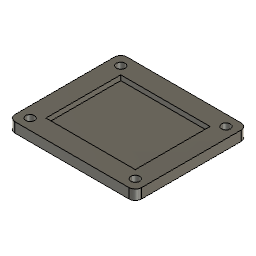
air_quality_sensor_holder (Autodesk Fusion 360 design; units mm, degrees)
Autodesk Fusion 360 part; units mm, degrees
sketch "Sketch10" plane through (0, 0, 0) normal (0, 0, 1) x (1, 0, 0)
  line L0 (0, 0) -> (45.72, 0)
  arc A0 (48.26, -2.54) -> (45.72, 0) centre (45.72, -2.54) ccw
  line L1 (45.72, -2.54) -> (48.26, -2.54) construction
  line L2 (45.72, -2.54) -> (45.72, 0) construction
  line L3 (48.26, -2.54) -> (48.26, -42.4361)
  arc A1 (48.26, -2.54) -> (45.72, 0) centre (45.72, -2.54) ccw
  arc A2 (45.72, -44.9761) -> (48.26, -42.4361) centre (45.72, -42.4361) ccw
  line L4 (0, -42.4361) -> (-2.54, -42.4361) construction
  line L5 (45.72, -44.9761) -> (0, -44.9761)
  arc A3 (-2.54, -42.4361) -> (0, -44.9761) centre (0, -42.4361) ccw
  arc A4 (-2.54, -42.4361) -> (0, -44.9761) centre (0, -42.4361) ccw
  line L6 (0, -42.4361) -> (0, -44.9761) construction
  arc A5 (0, 0) -> (-2.54, -2.54) centre (0, -2.54) ccw
  line L7 (-2.54, -42.4361) -> (-2.54, -2.54)
  point P0 (45.72, -44.9761)
  dimension "d5" = 45.72
  dimension "d7" = 2.54
  dimension "d8" = 90
  dimension "d9" = 39.8961
  dimension "d10" = 2.54
  dimension "d11" = 2.54
  dimension "d12" = 45.72
  dimension "d13" = 2.54
  dimension "d14" = 90
  dimension "d15" = 39.8961
  dimension "d16" = 2.54
  dimension "d17" = 2.54
  constraint coincident L0.start A5.start
  constraint horizontal L0
  constraint perpendicular L1 L3
  constraint coincident P0 A2.start
  constraint perpendicular L4 L7
  measures "d5" distance of L0.start L0.end
  measures "d7" radius of A0
  measures "d8" angle of L1 L2
  measures "d9" distance of A0.start L3.end
  measures "d10" radius of A1
  measures "d11" radius of A2
  measures "d12" distance of P0 L5.end
  measures "d13" radius of A4
  measures "d14" angle of L4 L6
  measures "d15" distance of L4.end A5.end
  measures "d16" radius of A3
  measures "d17" radius of A5
extrude "Extrude3" add sketch "Sketch10" along normal blind 4
sketch "Sketch11" plane through (0, 0, 4) normal (0, 0, 1) x (-1, 0, 0)
  arc A0 (-45.72, 44.9761) -> (-48.26, 42.4361) centre (-45.72, 42.4361) ccw
  line L0 (-48.26, 42.4361) -> (-48.26, 2.54)
  arc A1 (-48.26, 2.54) -> (-45.72, 0) centre (-45.72, 2.54) ccw
  line L1 (-45.72, 0) -> (0, 0)
  arc A2 (0, 0) -> (2.54, 2.54) centre (0, 2.54) ccw
  line L2 (2.54, 2.54) -> (2.54, 42.4361)
  arc A3 (2.54, 42.4361) -> (0, 44.9761) centre (0, 42.4361) ccw
  line L3 (0, 44.9761) -> (-45.72, 44.9761)
  circle A4 centre (-1.778, 4.318) radius 1.75
  dimension "d22" = 3.5
  measures "d22" diameter of A4
extrude "Extrude4" cut sketch "Sketch11" against normal blind 4 contours A4
sketch "Sketch12" plane through (0, 0, 4) normal (0, 0, 1) x (-1, 0, 0)
  circle A0 centre (-1.778, 4.318) radius 1.75
  arc A1 (-45.72, 44.9761) -> (-48.26, 42.4361) centre (-45.72, 42.4361) ccw
  line L0 (-48.26, 42.4361) -> (-48.26, 2.54)
  arc A2 (-48.26, 2.54) -> (-45.72, 0) centre (-45.72, 2.54) ccw
  line L1 (-45.72, 0) -> (0, 0)
  arc A3 (0, 0) -> (2.54, 2.54) centre (0, 2.54) ccw
  line L2 (2.54, 2.54) -> (2.54, 42.4361)
  arc A4 (2.54, 42.4361) -> (0, 44.9761) centre (0, 42.4361) ccw
  line L3 (0, 44.9761) -> (-45.72, 44.9761)
  circle A5 centre (-43.942, 4.318) radius 1.75
  dimension "d27" = 3.5
  measures "d27" diameter of A5
extrude "Extrude5" cut sketch "Sketch12" against normal blind 4 contours A5
sketch "Sketch13" plane through (0, 0, 4) normal (0, 0, 1) x (-1, 0, 0)
  circle A0 centre (-43.942, 4.318) radius 1.75
  circle A1 centre (-1.778, 4.318) radius 1.75
  arc A2 (-45.72, 44.9761) -> (-48.26, 42.4361) centre (-45.72, 42.4361) ccw
  line L0 (-48.26, 42.4361) -> (-48.26, 2.54)
  arc A3 (-48.26, 2.54) -> (-45.72, 0) centre (-45.72, 2.54) ccw
  line L1 (-45.72, 0) -> (0, 0)
  arc A4 (0, 0) -> (2.54, 2.54) centre (0, 2.54) ccw
  line L2 (2.54, 2.54) -> (2.54, 42.4361)
  arc A5 (2.54, 42.4361) -> (0, 44.9761) centre (0, 42.4361) ccw
  line L3 (0, 44.9761) -> (-45.72, 44.9761)
  circle A6 centre (-1.778, 40.6581) radius 1.75
  dimension "d32" = 3.5
  measures "d32" diameter of A6
extrude "Extrude6" cut sketch "Sketch13" against normal blind 4 contours A6
sketch "Sketch14" plane through (0, 0, 4) normal (0, 0, 1) x (-1, 0, 0)
  circle A0 centre (-1.778, 40.6581) radius 1.75
  circle A1 centre (-43.942, 4.318) radius 1.75
  circle A2 centre (-1.778, 4.318) radius 1.75
  arc A3 (-45.72, 44.9761) -> (-48.26, 42.4361) centre (-45.72, 42.4361) ccw
  line L0 (-48.26, 42.4361) -> (-48.26, 2.54)
  arc A4 (-48.26, 2.54) -> (-45.72, 0) centre (-45.72, 2.54) ccw
  line L1 (-45.72, 0) -> (0, 0)
  arc A5 (0, 0) -> (2.54, 2.54) centre (0, 2.54) ccw
  line L2 (2.54, 2.54) -> (2.54, 42.4361)
  arc A6 (2.54, 42.4361) -> (0, 44.9761) centre (0, 42.4361) ccw
  line L3 (0, 44.9761) -> (-45.72, 44.9761)
  circle A7 centre (-43.942, 40.6581) radius 1.75
  dimension "d37" = 3.5
  measures "d37" diameter of A7
extrude "Extrude7" cut sketch "Sketch14" against normal blind 4 contours A7
sketch "Sketch15" plane through (0, 0, 4) normal (0, 0, 1) x (-1, 0, 0)
  circle A0 centre (-43.942, 40.6581) radius 1.75
  circle A1 centre (-1.778, 40.6581) radius 1.75
  circle A2 centre (-43.942, 4.318) radius 1.75
  circle A3 centre (-1.778, 4.318) radius 1.75
  arc A4 (-45.72, 44.9761) -> (-48.26, 42.4361) centre (-45.72, 42.4361) ccw
  line L0 (-48.26, 42.4361) -> (-48.26, 2.54)
  arc A5 (-48.26, 2.54) -> (-45.72, 0) centre (-45.72, 2.54) ccw
  line L1 (-45.72, 0) -> (0, 0)
  arc A6 (0, 0) -> (2.54, 2.54) centre (0, 2.54) ccw
  line L2 (2.54, 2.54) -> (2.54, 42.4361)
  arc A7 (2.54, 42.4361) -> (0, 44.9761) centre (0, 42.4361) ccw
  line L3 (0, 44.9761) -> (-45.72, 44.9761)
  line L4 (-4.96, 7.5) -> (-40.76, 7.5)
  line L5 (-40.76, 7.5) -> (-40.76, 37.4761)
  line L6 (-40.76, 37.4761) -> (-4.96, 37.4761)
  line L7 (-4.96, 37.4761) -> (-4.96, 7.5)
  constraint horizontal L4
  constraint vertical L5
  constraint horizontal L6
  constraint vertical L7
extrude "Extrude8" cut sketch "Sketch15" against normal blind 2 contours L4 L5 L6 L7
